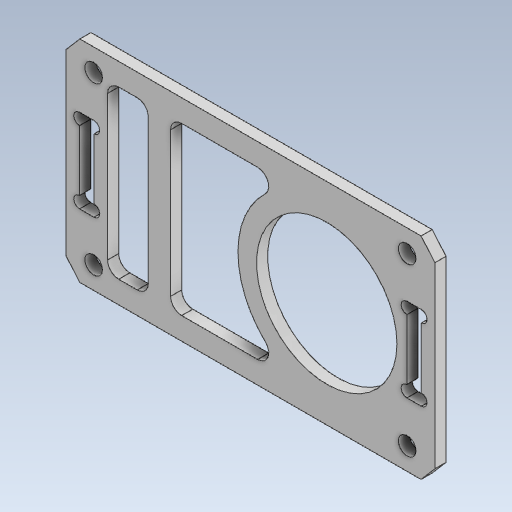
# Autodesk Inventor part: Trunk_neck_lower_frame
Saved by Autodesk Inventor 2020.4 (Build 244396000, 396)
## iProperties
Created: 2022-01-13
Part Number: Trunk_neck_lower_frame
Material: 一般
Document SubType Name: Modeling
Designer: Masato Kubotera
Density: 1 g/cm^3
Appearance: 既定
Description: A2017 T2
Author: Masato Kubotera
Autodesk Inventor part; units mm, degrees
ref_plane "YZ Plane" through (0, 0, 0) normal (1, 0, 0) x (0, 1, 0)
ref_plane "XZ Plane" through (0, 0, 0) normal (0, 1, 0) x (-1, 0, 0)
ref_plane "XY Plane" through (0, 0, 0) normal (0, 0, 1) x (1, 0, 0)
derived "Trunk_neck_Upper_frame.ipt"
sketch "スケッチ1" plane through (0, 0, 0) normal (0, 0, 1) x (1, 0, 0)
  circle A0 centre (0, 0) radius 10.5 construction
  line L0 (-28, -13.5) -> (-1, -13.5) construction
  line L1 (-1, -13.5) -> (-1, 13.5) construction
  line L2 (-1, 13.5) -> (-28, 13.5) construction
  line L3 (-28, 13.5) -> (-28, -13.5) construction
  line L4 (-28, -13.5) -> (-1, 13.5) construction
  line L5 (-1, -13.5) -> (-28, 13.5) construction
  line L6 (-31, -16) -> (12, -16) construction
  line L7 (12, -16) -> (12, 16) construction
  line L8 (12, 16) -> (-31, 16) construction
  line L9 (-31, 16) -> (-31, -16) construction
  line L10 (-31, -16) -> (12, 16) construction
  line L11 (12, -16) -> (-31, 16) construction
  line L12 (-31, -14.4) -> (-39.5, -14.4) construction
  line L13 (-39.5, -14.4) -> (-39.5, 14.4) construction
  line L14 (-39.5, 0) -> (12, 0) construction
  line L15 (-31, 14.4) -> (-39.5, 14.4) construction
  circle A1 centre (-1, -13.5) radius 1.35
  line L16 (-14.5, -13.5) -> (-14.5, 13.5) construction
  circle A2 centre (-28, -13.5) radius 1.35
  circle A3 centre (-1, 13.5) radius 1.35
  circle A4 centre (-28, 13.5) radius 1.35
  line L17 (14.5, -7.5) -> (17, -7.5) construction
  line L18 (17, -7.5) -> (17, 7.5) construction
  line L19 (17, 7.5) -> (14.5, 7.5) construction
  line L20 (14.5, 7.5) -> (14.5, -7.5) construction
  line L21 (14.5, -7.5) -> (17, 7.5) construction
  line L22 (17, -7.5) -> (14.5, 7.5) construction
  line L23 (14.45, 7.55) -> (17.05, 7.55)
  line L24 (17.05, 5.45) -> (17.05, -5.45)
  line L25 (17.05, -7.55) -> (14.45, -7.55)
  line L26 (14.45, -5.45) -> (14.45, 5.45)
  line L27 (14.45, 7.55) -> (17.05, -7.55) construction
  line L28 (17.05, 7.55) -> (14.45, -7.55) construction
  arc A5 (14.45, -5.45) -> (14.45, -7.55) centre (14.45, -6.5) ccw
  line L29 (15.75, -7.5) -> (15.75, 7.5) construction
  arc A6 (14.45, 7.55) -> (14.45, 5.45) centre (14.45, 6.5) ccw
  arc A7 (17.05, -7.55) -> (17.05, -5.45) centre (17.05, -6.5) ccw
  arc A8 (17.05, 5.45) -> (17.05, 7.55) centre (17.05, 6.5) ccw
  line L30 (-13.75, -16) -> (-13.75, 16) construction
  line L31 (-41.95, -5.45) -> (-41.95, 5.45)
  line L32 (-44.55, 5.45) -> (-44.55, -5.45)
  line L33 (-42, 7.5) -> (-42, -7.5) construction
  line L34 (-43.25, -7.5) -> (-43.25, 7.5) construction
  line L35 (-44.5, -7.5) -> (-44.5, 7.5) construction
  line L36 (-42, -7.5) -> (-44.5, 7.5) construction
  line L37 (-44.5, -7.5) -> (-42, 7.5) construction
  line L38 (-44.55, 7.55) -> (-41.95, -7.55) construction
  line L39 (-41.95, 7.55) -> (-44.55, -7.55) construction
  arc A9 (-41.95, 5.45) -> (-41.95, 7.55) centre (-41.95, 6.5) ccw
  line L40 (-44.5, 7.5) -> (-42, 7.5) construction
  line L41 (-41.95, 7.55) -> (-44.55, 7.55)
  line L42 (-42, -7.5) -> (-44.5, -7.5) construction
  line L43 (-44.55, -7.55) -> (-41.95, -7.55)
  arc A10 (-41.95, -7.55) -> (-41.95, -5.45) centre (-41.95, -6.5) ccw
  arc A11 (-44.55, -5.45) -> (-44.55, -7.55) centre (-44.55, -6.5) ccw
  arc A12 (-44.55, 7.55) -> (-44.55, 5.45) centre (-44.55, 6.5) ccw
  circle A13 centre (14.5, -15) radius 1.6
  circle A14 centre (14.5, 15) radius 1.6
  circle A15 centre (-42, 15) radius 1.6
  circle A16 centre (-42, -15) radius 1.6
  line L44 (12, -60.5) -> (17, -60.5) construction
  line L45 (17, -60.5) -> (17, 60.5) construction
  line L46 (17, 60.5) -> (12, 60.5) construction
  line L47 (12, -60.5) -> (17, 60.5) construction
  line L48 (17, -60.5) -> (12, 60.5) construction
  arc A17 (-5.5678, 15) -> (-5.5678, -15) centre (0, 0) ccw
  line L49 (-3.65, -16) -> (1.65, -16) construction
  line L50 (1.65, -16) -> (1.65, 16) construction
  line L51 (1.65, 16) -> (-3.65, 16) construction
  line L52 (-3.65, 16) -> (-3.65, -16) construction
  line L53 (-3.65, -16) -> (1.65, 16) construction
  line L54 (1.65, -16) -> (-3.65, 16) construction
  line L55 (-44.5, 60.5) -> (-39.5, 60.5) construction
  line L56 (-44.5, -60.5) -> (-44.5, 60.5) construction
  line L57 (-39.5, 60.5) -> (-39.5, -60.5) construction
  line L58 (-39.5, -60.5) -> (-44.5, -60.5) construction
  line L59 (12, -60.5) -> (12, 60.5) construction
  arc A18 (0.9585, -11.7148) -> (-2.6741, -11.4457) centre (-1, -13.5) ccw
  arc A19 (2.8942, -12.3145) -> (2.8942, 12.3145) centre (0, 0) ccw
  arc A20 (-2.6741, 11.4457) -> (0.9585, 11.7148) centre (-1, 13.5) ccw
  arc A21 (-4.677, -11.7537) -> (-2.6741, -11.4457) centre (-3.9375, -9.8954) ccw
  arc A22 (0.9585, -11.7148) -> (2.8942, -12.3145) centre (2.4366, -10.3675) ccw
  arc A23 (2.8942, 12.3145) -> (0.9585, 11.7148) centre (2.4366, 10.3675) ccw
  arc A24 (-2.6741, 11.4457) -> (-4.677, 11.7537) centre (-3.9375, 9.8954) ccw
  arc A25 (0.9585, 11.7148) -> (-2.6741, 11.4457) centre (-1, 13.5) ccw
  arc A26 (-2.6741, -11.4457) -> (0.9585, -11.7148) centre (-1, -13.5) ccw
  arc A27 (-4.677, 11.7537) -> (-4.677, -11.7537) centre (0, 0) ccw
  circle A28 centre (14.5, -15) radius 3
  circle A29 centre (14.5, 15) radius 3
  line L60 (-25.8154, -15) -> (-5.5678, -15)
  line L61 (-39.5, -15) -> (-32.15, -15)
  line L62 (-32.15, -15) -> (-32.15, 15)
  line L63 (-32.15, 15) -> (-39.5, 15)
  line L64 (-39.5, 15) -> (-39.5, -15)
  line L65 (-39.5, -15) -> (-32.15, 15) construction
  line L66 (-32.15, -15) -> (-39.5, 15) construction
  line L67 (-44.5, -19) -> (17, -19)
  line L68 (-28.15, -10.8542) -> (-28.15, 10.8542)
  line L69 (-44.5, 19) -> (17, 19)
  circle A30 centre (-28, -13.5) radius 2.65
  circle A31 centre (-28, 13.5) radius 2.65
  line L70 (17, -19) -> (19.5, -16.0779)
  line L71 (19.5, -16.0779) -> (19.5, 16.0779)
  line L72 (17, 19) -> (19.5, 16.0779)
  line L73 (-44.5, -19) -> (-47, -16.0779)
  line L74 (-47, -16.0779) -> (-47, 16.0779)
  line L75 (-44.5, 19) -> (-47, 16.0779)
  line L76 (-25.8154, 15) -> (-5.5678, 15)
  point P0 (-14.5, 0)
  point P1 (-9.5, 0)
  point P2 (-14.5, 0)
  point P3 (15.75, 0)
  point P4 (15.75, 0)
  point P5 (15.75, 0)
  point P6 (15.75, 0)
  point P7 (-43.25, 0)
  point P8 (-43.25, 0)
  point P9 (-43.25, 0)
  point P10 (-43.25, 0)
  point P11 (14.5, 0)
  point P12 (14.5, 0)
  point P13 (-1, 0)
  point P14 (-35.825, 0)
sketch "スケッチ2" plane through (0, 0, 0) normal (0, 0, 1) x (1, 0, 0)
  circle A0 centre (0, 0) radius 12.65
  arc A1 (-4.677, 11.7537) -> (-4.677, -11.7537) centre (0, 0) ccw projected
  line L0 (-25.8154, 15) -> (-5.5678, 15) projected
  line L1 (-28.15, -10.8542) -> (-28.15, 10.8542) projected
  line L2 (-25.8154, -15) -> (-5.5678, -15) projected
  line L3 (-28.15, 0) -> (-28.15, 15)
  line L4 (-28.15, 15) -> (-5.5678, 15)
  line L5 (-39.5, 0) -> (12, 0) construction
  line L6 (-28.15, 0) -> (-28.15, -15)
  line L7 (-28.15, -15) -> (-5.5678, -15)
  line L8 (-44.5, 19) -> (17, 19) projected
  line L9 (-44.5, 19) -> (-47, 16.0779) projected
  line L10 (-47, -16.0779) -> (-47, 16.0779) projected
  line L11 (-44.5, -19) -> (-47, -16.0779) projected
  line L12 (-44.5, -19) -> (17, -19) projected
  line L13 (17, -19) -> (19.5, -16.0779) projected
  line L14 (19.5, -16.0779) -> (19.5, 16.0779) projected
  line L15 (17, 19) -> (19.5, 16.0779) projected
  circle A2 centre (14.5, 15) radius 1.6 projected
  circle A3 centre (14.5, -15) radius 1.6 projected
  circle A4 centre (-42, -15) radius 1.6 projected
  circle A5 centre (-42, 15) radius 1.6 projected
  arc A6 (-41.95, 5.45) -> (-41.95, 7.55) centre (-41.95, 6.5) ccw projected
  line L16 (-41.95, -5.45) -> (-41.95, 5.45) projected
  line L17 (-41.95, 7.55) -> (-44.55, 7.55) projected
  arc A7 (-44.55, 7.55) -> (-44.55, 5.45) centre (-44.55, 6.5) ccw projected
  line L18 (-44.55, 5.45) -> (-44.55, -5.45) projected
  arc A8 (-44.55, -5.45) -> (-44.55, -7.55) centre (-44.55, -6.5) ccw projected
  line L19 (-44.55, -7.55) -> (-41.95, -7.55) projected
  arc A9 (-41.95, -7.55) -> (-41.95, -5.45) centre (-41.95, -6.5) ccw projected
  line L20 (17.05, -7.55) -> (14.45, -7.55) projected
  arc A10 (14.45, -5.45) -> (14.45, -7.55) centre (14.45, -6.5) ccw projected
  line L21 (14.45, -5.45) -> (14.45, 5.45) projected
  arc A11 (14.45, 7.55) -> (14.45, 5.45) centre (14.45, 6.5) ccw projected
  line L22 (14.45, 7.55) -> (17.05, 7.55) projected
  arc A12 (17.05, 5.45) -> (17.05, 7.55) centre (17.05, 6.5) ccw projected
  line L23 (17.05, 5.45) -> (17.05, -5.45) projected
  arc A13 (17.05, -7.55) -> (17.05, -5.45) centre (17.05, -6.5) ccw projected
  arc A14 (-5.5678, 15) -> (-5.5678, -15) centre (0, 0) ccw projected
  line L24 (-39.5, 15) -> (-32.15, 15)
  line L25 (-32.15, 15) -> (-32.15, -15)
  line L26 (-32.15, -15) -> (-39.5, -15)
  line L27 (-39.5, -15) -> (-39.5, 15)
  point P0 (-28.15, 10.8542)
  dimension "d1" = 12.65
  dimension "d2" = 25.3
  constraints: 16 end point, 2 parallel, 1 centre point, 1 coincident, 1 collinear, 1 horizontal, 1 midpoint, 1 perpendicular, 1 point on line, 1 symmetric about line
  measures "d1" radius of A1
  measures "d2" diameter of A0
extrude "押し出し1" add sketch "スケッチ2" along normal blind 2
fillet "フィレット1" radius 2 8 edges at (-39.5, -15, 1) (-39.5, 15, 1) (-32.15, 15, 1) (-28.15, 15, 1) (-28.15, -15, 1) (-32.15, -15, 1) (-5.5678, -15, 1) (-5.5678, 15, 1)
equation "\"d2\" = 2 * d1"
